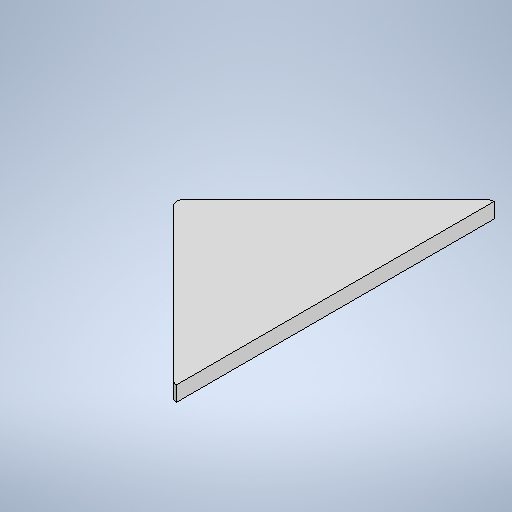
# Autodesk Inventor part: MNT-CDF-605 CAP
Saved by Autodesk Inventor 2025 (Build 290162010, 162A)
## iProperties
Created: 2025-01-16
Part Number: MNT-CDF-605 CAP
Material: Stainless Steel
Document SubType Name: Sheet Metal
Designer: pokla
Density: 8 g/cm^3
Sheet Metal Rule: AISI304 2mm Die16
Appearance: Default
Author: pokla
Autodesk Inventor part; units mm, degrees
ref_plane "YZ Plane" through (0, 0, 0) normal (1, 0, 0) x (0, 1, 0)
ref_plane "XZ Plane" through (0, 0, 0) normal (0, 1, 0) x (-1, 0, 0)
ref_plane "XY Plane" through (0, 0, 0) normal (0, 0, 1) x (1, 0, 0)
sketch "Sketch1" plane through (0, 0, 0) normal (0, 0, 1) x (1, 0, 0)
  line L0 (-20.5, 21) -> (20.5, 21)
  line L1 (20.5, 21) -> (20.5, -21)
  line L2 (20.5, -21) -> (-20.5, -21)
  line L3 (-20.5, -21) -> (-20.5, 21) construction
  line L4 (-20.5, 21) -> (20.5, -21) construction
  line L5 (-20.5, -21) -> (-41.5, 0)
  line L6 (-41.5, 0) -> (-20.5, 21)
  point P0 (0, 0)
  point P1 (0, 0)
  point P2 (20.5, 0)
  dimension "d0" = 41
  dimension "d1" = 42
  dimension "d4" = 62
  measures "d0" distance of L0.start L0.end
  measures "d1" distance of L2.end L0.start
  measures "d4" distance of point (20.5, 0) L5.end
extrude "Plate1" add sketch "Sketch1" along normal blind 2
fillet "Corner Round2" radius 1 3 edges at (-20.5, -21, 1) (-41.5, 0, 1) (-20.5, 21, 1)
sketch "Sketch2" plane through (0, 0, 2) normal (0, 0, 1) x (1, 0, 0)
  arc A0 (-20.7929, -20.7071) -> (-20.0858, -21) centre (-20.0858, -20) ccw projected
  line L0 (-40.7929, 0.7071) -> (-20.7929, 20.7071) projected
  line L1 (20.5, -21) -> (-20.0858, -21) projected
  line L2 (20.5, 21) -> (20.5, -21) projected
  line L3 (-20.0858, 21) -> (20.5, 21) projected
  arc A1 (-20.0858, 21) -> (-20.7929, 20.7071) centre (-20.0858, 20) ccw projected
  arc A2 (-20.7929, -20.7071) -> (-20.0858, -21) centre (-20.0858, -20) ccw projected
  arc A3 (-20.0858, 21) -> (-20.7929, 20.7071) centre (-20.0858, 20) ccw projected
  line L4 (-20.0858, -21) -> (-20.0858, 21)
  point P0 (0, 0)
  constraints: 2 end point, 1 vertical
extrude "Extrusion1" cut sketch "Sketch2" against normal through all
equation "\"d2\" = Thickness"
equation "\"BendReliefWidth\" = Thickness"
equation "\"BendReliefDepth\" = 0.5 * Thickness"
equation "\"CornerReliefSize\" = 4 * Thickness"
equation "\"MinimumRemnant\" = 2 * Thickness"
equation "\"TransitionRadius\" = BendRadius"
equation "\"JacobiRadiusSize\" = BendRadius"
equation "\"GapSize\" = Thickness"
equation "\"Thickness\" = 2"
equation "\"BendRadius\" = 2.75"
body "Solid1"
